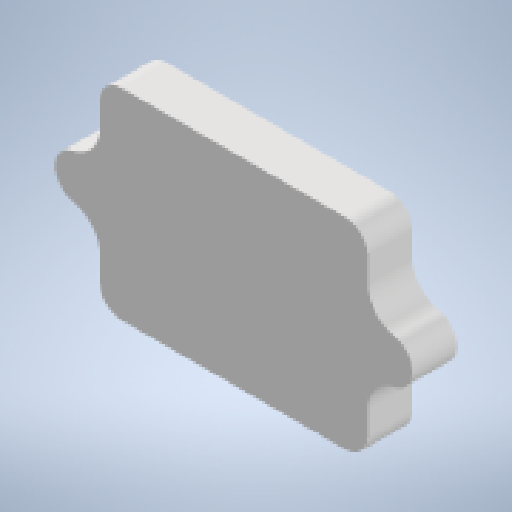
# Autodesk Inventor part: Deshumidicador
Saved by Autodesk Inventor 2024 (Build 280153000, 153)
## iProperties
Created: 2024-07-18
Part Number: Deshumidicador
Material: Genérico
Document SubType Name: Modeling
Designer: sergi
Density: 1 g/cm^3
Appearance: Valor por defecto
Author: sergi
Autodesk Inventor part; units mm, degrees
ref_plane "YZ Plane" through (0, 0, 0) normal (1, 0, 0) x (0, 1, 0)
ref_plane "XZ Plane" through (0, 0, 0) normal (0, 1, 0) x (-1, 0, 0)
ref_plane "XY Plane" through (0, 0, 0) normal (0, 0, 1) x (1, 0, 0)
sketch "Boceto1" plane through (0, 0, 0) normal (0, 0, 1) x (1, 0, 0)
  line L0 (-25, 22.5) -> (25, 22.5)
  line L1 (30, 17.5) -> (30, -17.5)
  line L2 (25, -22.5) -> (-25, -22.5)
  line L3 (-30, -17.5) -> (-30, 17.5)
  line L4 (-30, 22.5) -> (30, -22.5) construction
  line L5 (30, 22.5) -> (-30, -22.5) construction
  line L6 (-25, 20.5) -> (25, 20.5)
  line L7 (28, 17.5) -> (28, -17.5)
  line L8 (25, -20.5) -> (-25, -20.5)
  line L9 (-28, -17.5) -> (-28, 17.5)
  arc A0 (-30, -17.5) -> (-25, -22.5) centre (-25, -17.5) ccw
  arc A1 (25, -22.5) -> (30, -17.5) centre (25, -17.5) ccw
  arc A2 (30, 17.5) -> (25, 22.5) centre (25, 17.5) ccw
  arc A3 (-25, 22.5) -> (-30, 17.5) centre (-25, 17.5) ccw
  arc A4 (-25, 20.5) -> (-28, 17.5) centre (-25, 17.5) ccw
  arc A5 (28, 17.5) -> (25, 20.5) centre (25, 17.5) ccw
  arc A6 (25, -20.5) -> (28, -17.5) centre (25, -17.5) ccw
  arc A7 (-28, -17.5) -> (-25, -20.5) centre (-25, -17.5) ccw
  point P0 (0, 0)
  point P1 (-28, 20.5)
  point P2 (28, 20.5)
  point P3 (28, -20.5)
  point P4 (-28, -20.5)
  dimension "d0" = 45
  dimension "d1" = 2
  dimension "d5" = 5
  dimension "d6" = 3
  constraints: 20 end point, 16 point on circle, 16 point on line, 16 tangent, 8 centre point, 6 equal radius, 4 parallel, 2 midpoint, 2 perpendicular, 1 horizontal, 3 other
  measures "d0" distance of L5.start L4.end
  measures "d1" distance between parallel lines of L3 L9
  measures "d5" radius of A0
  measures "d6" radius of A4
extrude "Extrusión1" add sketch "Boceto1" along normal blind 10 contours L0 A2 L1 A1 L2 A0 L3 A3 | L6 A5 L7 A6 L8 A7 L9 A4
shell "Vaciado1" thickness 1 removed faces 1 at (-8.3333, -7.5, 0)
sketch "Boceto2" plane through (0, 0, 0) normal (0, 0, -1) x (-1, 0, 0)
  line L0 (25, -22.5) -> (-25, -22.5) projected
  arc A0 (-30, -17.5) -> (-25, -22.5) centre (-25, -17.5) ccw projected
  line L1 (-30, -17.5) -> (-30, 17.5) projected
  arc A1 (-25, 22.5) -> (-30, 17.5) centre (-25, 17.5) ccw projected
  line L2 (-25, 22.5) -> (25, 22.5) projected
  arc A2 (30, 17.5) -> (25, 22.5) centre (25, 17.5) ccw projected
  line L3 (30, 17.5) -> (30, -17.5) projected
  arc A3 (25, -22.5) -> (30, -17.5) centre (25, -17.5) ccw projected
  line L4 (30, 0) -> (40, 0)
  line L5 (-30, 0) -> (-40, 0)
  circle A4 centre (35, 0) radius 5
  circle A5 centre (-35, 0) radius 5
  circle A6 centre (35, 0) radius 2.1
  circle A7 centre (-35, 0) radius 2.1
  circle A8 centre (37.5, -12.2474) radius 7.5
  line L6 (30, 17.5) -> (30, -17.5) projected
  circle A9 centre (-37.5, 12.2474) radius 7.5
  circle A10 centre (-37.5, -12.2474) radius 7.5
  circle A11 centre (37.5, 12.2474) radius 7.5
  line L7 (-30, -17.5) -> (-30, 17.5) projected
  point P0 (0, 0)
  point P1 (-36, -4.899)
  point P2 (-30, -12.2474)
  point P3 (-30, 12.2474)
  point P4 (-36, 4.899)
  point P5 (36, 4.899)
  point P6 (30, 12.2474)
  point P7 (30, -12.2474)
  point P8 (36, -4.899)
  dimension "d8" = 10
  dimension "d9" = 10
  dimension "d10" = 4.2
  dimension "d11" = 4.2
  dimension "d12" = 15
  dimension "d14" = 15
  dimension "d15" = 15
  dimension "d16" = 15
  constraints: 6 centre point, 4 end point, 4 midpoint, 4 tangent, 2 coincident, 2 horizontal, 10 other
  measures "d8" distance of L4.start L4.end
  measures "d9" distance of L5.start L5.end
  measures "d10" diameter of A6
  measures "d11" diameter of A7
  measures "d12" diameter of A8
  measures "d14" diameter of A9
  measures "d15" diameter of A10
  measures "d16" diameter of A11
extrude "Extrusión2" add sketch "Boceto2" against normal blind 10 contours L3 A4 A8 | A10 A5 L1 | A4 L4 A6 | L3 A11 A4 | L4 A6 A4 | A5 A9 L1 | A5 L5 A7 | L5 A7 A5 | A6 L4 | L4 A6 | A7 L5 | L5 A7
sketch "Boceto3" plane through (0, 0, 0) normal (0, 0, -1) x (-1, 0, 0)
  arc A0 (-36, 4.899) -> (-36, -4.899) centre (-35, 0) ccw projected
  arc A1 (36, -4.899) -> (36, 4.899) centre (35, 0) ccw projected
  point P0 (0, 0)
  constraints: 2 coincident
hole "Agujero1" at (35, 0, 0) at (-35, 0, 0) direction (0, 0, 1) diameter 4.2 depth 7
